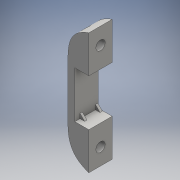
# Autodesk Inventor part: top_mount
Saved by Autodesk Inventor 2016 (Build 200138000, 138)
## iProperties
Created: 2017-06-06
Part Number: top_mount
Material: Ogólny
Document SubType Name: Modeling
Designer: Karol
Density: 1 g/cm^3
Appearance: Domyślna
Author: Karol
Autodesk Inventor part; units mm, degrees
sketch "Sketch1" plane through (0, 0, 0) normal (0, 1, 0) x (-1, 0, 0)
  line L0 (0, 0) -> (0, -5)
  line L1 (0, 0) -> (0, 5)
  line L2 (0, 5) -> (-3, 5)
  line L3 (0, -5) -> (-3, -5)
  line L4 (-3, 5) -> (-3, 13)
  line L5 (-3, -5) -> (-3, -13)
  line L6 (1.5, 0) -> (1.5, -5)
  line L7 (1.5, 0) -> (1.5, 5)
  spline S0 degree 3 poles (-3, 13) (1.5, 11.5121) (1.5, 8.2561) (1.5, 5) knots 0 0 0 0 1 1 1 1
  spline S1 degree 3 poles (-3, -13) (1.5, -11.5121) (1.5, -8.2561) (1.5, -5) knots 0 0 0 0 1 1 1 1
  point P0 (-3, 9)
  point P1 (-3, -9)
  dimension "d0" = 5
  dimension "d1" = 5
  dimension "d2" = 3
  dimension "d3" = 3
  dimension "d4" = 8
  dimension "d5" = 8
  dimension "d6" = 5
  dimension "d7" = 5
  constraints: 16 end point, 8 vertical, 2 horizontal, 2 midpoint, 4 other
  measures "d0" distance of L0.start L0.end
  measures "d1" distance of L0.start L1.end
  measures "d2" distance of L1.end L2.end
  measures "d3" distance of L0.end L3.end
  measures "d4" distance of L2.end L4.end
  measures "d5" distance of L3.end L5.end
  measures "d6" distance of L6.start L6.end
  measures "d7" distance of L6.start L7.end
extrude "Extrusion1" add sketch "Sketch1" along normal blind 5
sketch "Sketch2" plane through (3, 0, 13) normal (1, 0, 0) x (0, 0, -1)
  circle A0 centre (3.5513, 2.5007) radius 1
  line L0 (13, 0) -> (13, 5)
  line L1 (8, 5) -> (18, 5) projected
  line L2 (4.7093, 4.4988) -> (5.8606, 2.4969)
  line L3 (5.8606, 2.4969) -> (4.7026, 0.4988)
  line L4 (4.7026, 0.4988) -> (2.3933, 0.5026)
  line L5 (2.3933, 0.5026) -> (1.2419, 2.5045)
  line L6 (1.2419, 2.5045) -> (2.3999, 4.5026)
  line L7 (2.3999, 4.5026) -> (4.7093, 4.4988)
  point P0 (22, 2.5)
  dimension "d12" = 2
  dimension "d33" = 4
  constraints: 14 end point, 3 coincident, 1 centre point, 1 midpoint, 13 other
  measures "d12" diameter of A0
  measures "d33" distance between parallel lines of L7 L4
extrude "Extrusion2" cut sketch "Sketch2" against normal blind 2 contours A0
ref_plane "Work Plane3" through (1.5, 0, 13) normal (1, 0, 0) x (0, 0, -1)
sketch "Sketch3" plane through (1.5, 0, 13) normal (1, 0, 0) x (0, 0, -1)
  circle A0 centre (3.5513, 2.5007) radius 1 projected
  circle A1 centre (3.5513, 2.5007) radius 1 projected
  line L0 (0, 0) -> (8, 0) projected
  line L1 (8, 0) -> (8, 5) projected
  line L2 (0, 5) -> (8, 5) projected
  line L3 (0, 0) -> (0, 5) projected
  line L4 (2.3935, 0.5024) -> (1.2419, 2.5042) projected
  line L5 (1.2419, 2.5042) -> (2.3996, 4.5024) projected
  line L6 (2.3996, 4.5024) -> (4.709, 4.4989) projected
  line L7 (4.709, 4.4989) -> (5.8607, 2.4972) projected
  line L8 (5.8607, 2.4972) -> (4.7029, 0.4989) projected
  line L9 (4.7029, 0.4989) -> (2.3935, 0.5024) projected
  circle A2 centre (3.5513, 2.5007) radius 1 projected
  point P0 (13, 0)
extrude "Extrusion3" cut sketch "Sketch3" against normal blind 10 contours A0 | L4 L5 L6 L7 L8 L9
ref_plane "Work Plane5" through (3, 0, 0) normal (0, 0, 1) x (0, 1, 0)
mirror "Mirror1" about plane through (3, 0, 0) normal (0, 0, 1) of "Extrusion2", "Extrusion3"
ref_plane "Work Plane6" through (0, 1.1, 0) normal (0, -1, 0) x (1, 0, 0)
sketch "Sketch5" plane through (0, 1.1, 0) normal (0, -1, 0) x (1, 0, 0)
  line L0 (3, 5) -> (0, 5) projected
  line L1 (0, 5) -> (0, -5) projected
  line L2 (1, 5) -> (0, 4)
  line L3 (0, -5) -> (3, -5) projected
  line L4 (1, -5) -> (0, -4)
  point P0 (0, 0)
  constraints: 4 end point, 4 point on line
extrude "Extrusion4" add sketch "Sketch5" against normal blind 0.5
ref_plane "Work Plane7" through (0, 4.9, 0) normal (0, 1, 0) x (1, 0, 0)
sketch "Sketch6" plane through (0, 4.9, 0) normal (0, 1, 0) x (1, 0, 0)
  line L0 (1, -5) -> (0, -5) projected
  line L1 (1, -5) -> (0, -4) projected
  line L2 (0, -5) -> (0, -4) projected
  line L3 (0, 4) -> (0, 5) projected
  line L4 (0, 4) -> (1, 5) projected
  line L5 (0, 5) -> (1, 5) projected
  point P0 (0, 0)
extrude "Extrusion5" add sketch "Sketch6" against normal blind 0.5
body "Solid1"
